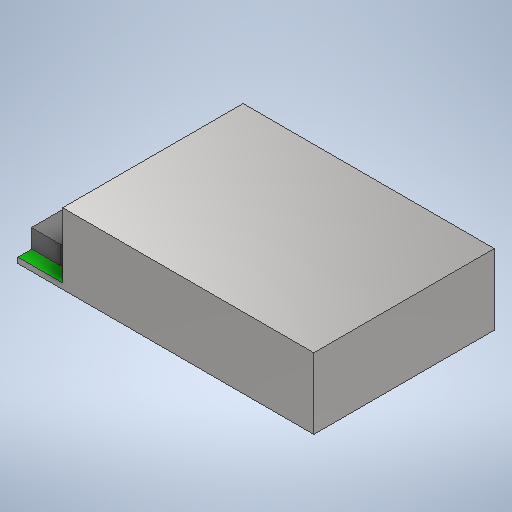
# Autodesk Inventor part: power supply
Saved by Autodesk Inventor 2025.1 (Build 291241000, 241)
## iProperties
Created: 2024-10-28
Part Number: power supply
Material: 일반
Document SubType Name: Modeling
Designer: gmsee
Density: 1 g/cm^3
Appearance: 기본값
Author: gmsee
Autodesk Inventor part; units mm, degrees
ref_plane "YZ Plane" through (0, 0, 0) normal (1, 0, 0) x (0, 1, 0)
ref_plane "XZ Plane" through (0, 0, 0) normal (0, 1, 0) x (-1, 0, 0)
ref_plane "XY Plane" through (0, 0, 0) normal (0, 0, 1) x (1, 0, 0)
sketch "스케치2" plane through (0, 0, 0) normal (0, 1, 0) x (-1, 0, 0)
  line L0 (55.5, -48.5) -> (-79.5, -48.5)
  line L1 (-79.5, -48.5) -> (-79.5, 48.5)
  line L2 (-79.5, 48.5) -> (55.5, 48.5)
  line L3 (55.5, 48.5) -> (55.5, -48.5)
  point P0 (0, 0)
  dimension "d6" = 79.5
  dimension "d7" = 48.5
  dimension "d8" = 48.5
  dimension "d9" = 55.5
  constraints: 8 end point, 2 parallel, 1 horizontal, 1 perpendicular
  measures "d6" distance from line of point (0, 0) L1
  measures "d7" distance from line of L0 point (0, 0)
  measures "d8" distance from line of L2 point (0, 0)
  measures "d9" distance from line of point (0, 0) L3
extrude "돌출2" add sketch "스케치2" along normal blind 38
sketch "스케치4" plane through (0, 0, 0) normal (0, 1, 0) x (-1, 0, 0)
  line L0 (-79.5, -48.5) -> (55.5, -48.5) projected
  line L1 (55.5, -48.5) -> (79.5, -48.5)
  line L2 (79.5, -48.5) -> (79.5, 48.5)
  line L3 (79.5, 48.5) -> (55.5, 48.5)
  line L4 (55.5, 48.5) -> (55.5, -48.5)
  point P0 (0, 0)
  dimension "d14" = 24
  constraints: 8 end point, 2 parallel, 1 horizontal, 1 perpendicular
  measures "d14" distance between parallel lines of L4 L2
extrude "돌출4" add sketch "스케치4" along normal blind 3
sketch "스케치5" plane through (0, 3, 0) normal (0, 1, 0) x (1, 0, 0)
  line L0 (-79.6369, 26.9038) -> (-63.7841, 26.9038)
  line L1 (-63.7841, 26.9038) -> (-63.7841, -41.096)
  line L2 (-63.7841, -41.096) -> (-79.6369, -41.096)
  line L3 (-79.6369, -41.096) -> (-79.6369, 26.9038)
  point P0 (0, 0)
  constraints: 8 end point, 2 parallel, 1 horizontal, 1 perpendicular
extrude "돌출5" add sketch "스케치5" along normal blind 10
